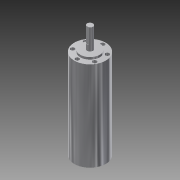
# Autodesk Inventor part: Motor
Saved by Autodesk Inventor 2015 (Build 190159000, 159)
## iProperties
Created: 2016-09-19
Part Number: Motor
Material: Generic
Document SubType Name: Modeling
Designer: James Yelland
Density: 1 g/cm^3
Appearance: Default
Author: James Yelland
Autodesk Inventor part; units mm, degrees
ref_plane "YZ Plane" through (0, 0, 0) normal (1, 0, 0) x (0, 1, 0)
ref_plane "XY Plane" through (0, 0, 0) normal (0, 0, 1) x (1, 0, 0)
sketch "Sketch1" plane through (0, 0, 0) normal (0, 0, 1) x (1, 0, 0)
  circle A0 centre (0, 0) radius 8
  dimension "d0" = 16
  constraints: 1 centre point, 1 coincident
  measures "d0" diameter of A0
extrude "Extrusion1" add sketch "Sketch1" along normal blind 45.7
sketch "Sketch2" plane through (0, 0, 45.7) normal (0, 0, 1) x (1, 0, 0)
  circle A0 centre (0, 6.5) radius 1
  circle A1 centre (5.6292, 3.25) radius 1
  circle A2 centre (5.6292, -3.25) radius 1
  circle A3 centre (0, -6.5) radius 1
  circle A4 centre (-5.6292, -3.25) radius 1
  circle A5 centre (-5.6292, 3.25) radius 1
  point P0 (0, 0)
  point P1 (0, 0)
  dimension "d5" = 2
  dimension "d8" = 360
  constraints: 6 centre point, 13 other
  measures "d5" diameter of A0
extrude "Extrusion2" cut sketch "Sketch2" against normal blind 10
sketch "Sketch3" plane through (0, 0, 45.7) normal (0, 0, 1) x (1, 0, 0)
  circle A0 centre (0, 0) radius 5
  dimension "d12" = 10
  constraints: 1 centre point, 1 coincident
  measures "d12" diameter of A0
extrude "Extrusion3" add sketch "Sketch3" along normal blind 1.1
sketch "Sketch8" plane through (0, 0, 46.8) normal (0, 0, 1) x (1, 0, 0)
  circle A0 centre (0, 0) radius 1.5
  dimension "d31" = 3
  constraints: 1 centre point, 1 coincident
  measures "d31" diameter of A0
extrude "Extrusion8" add sketch "Sketch8" along normal blind 10.65
ref_plane "Work Plane5" through (0, -1.5, 46.8) normal (0, 1, 0) x (-1, 0, 0)
sketch "Sketch9" plane through (0, -1.5, 46.8) normal (0, 1, 0) x (-1, 0, 0)
  line L0 (1.5, 10.65) -> (-1.5, 10.65) projected
  line L1 (0, 10.65) -> (1.5, 10.65)
  line L2 (1.5, 10.65) -> (1.5, 2.85)
  line L3 (1.5, 2.85) -> (-1.5, 2.85)
  line L4 (-1.5, 2.85) -> (-1.5, 10.65)
  line L5 (-1.5, 10.65) -> (0, 10.65)
  point P0 (0, -46.8)
  dimension "d34" = 1.5
  dimension "d35" = 7.8
  constraints: 10 end point, 3 perpendicular, 2 point on line, 1 collinear, 1 midpoint
  measures "d34" distance of L1.start L1.end
  measures "d35" distance of L1.end L2.end
extrude "Extrusion9" cut sketch "Sketch9" along normal blind 0.2
body "Solid1"
